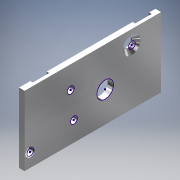
# Autodesk Inventor part: OslonaLewejPrzekladni
Saved by Autodesk Inventor 2019 (Build 230136000, 136)
## iProperties
Created: 2022-03-16
Part Number: OslonaLewejPrzekladni
Material: Aluminium 6061
Document SubType Name: Modeling
Designer: Michał
Density: 2.7 g/cm^3
Appearance: Aluminium — płaski
Mass: 6.40731 g
Surface Area: 27.93 cm^2
Volume: 2.37308 cm^3
Author: Michał
Autodesk Inventor part; units mm, degrees
ref_plane "YZ Plane" through (0, 0, 0) normal (1, 0, 0) x (0, 1, 0)
sketch "Szkic1" plane through (0, 0, 0) normal (1, 0, 0) x (0, 1, 0)
  line L0 (0, 0) -> (25, 0)
  line L1 (25, 0) -> (25, -49)
  line L2 (25, -49) -> (0, -49)
  line L3 (0, -49) -> (0, 0)
  dimension "d0" = 25
  dimension "d1" = 49
  constraints: 8 end point, 2 parallel, 1 horizontal, 1 perpendicular
  measures "d0" distance of L0.start L0.end
  measures "d1" distance of L0.end L1.end
extrude "Wyciągnięcie proste1" add sketch "Szkic1" along normal blind 2
sketch "Szkic2" plane through (2, 0, 0) normal (1, 0, 0) x (0, 0, -1)
  circle A0 centre (28.9, 11) radius 3
  circle A1 centre (17.6791, 7.0925) radius 1.25
  circle A2 centre (16.5416, 17.0276) radius 1.25
  circle A3 centre (2, 5) radius 1.2295
  circle A4 centre (38.5, 20) radius 1.2295
  constraints: 5 centre point, 10 other
hole "Otwór1" at (2, 5, -2) direction (-1, 0, 0) diameter 3.4 end through all clearance for "Śruba ze łbem stożkowym ISO 2009/7046" size "M3" standard "ISO"
hole "Otwór2" at (2, 20, -38.5) direction (-1, 0, 0) diameter 3.4 end through all countersink diameter 6.3 countersink angle 90 clearance for "Śruba ze łbem stożkowym ISO 2009/7046" size "M3" standard "ISO"
extrude "Wyciągnięcie proste2" cut sketch "Szkic2" against normal through all contours A0 | A1 | A2
sketch "Szkic3" plane through (0, 25, 0) normal (0, 1, 0) x (1, 0, 0)
  line L0 (0, 4.05) -> (-5, 4.05)
  line L1 (-5, 46.7) -> (0, 46.7)
  line L2 (0, 40.8) -> (-5, 40.8)
  line L3 (0, 4.05) -> (0.9, 4.05)
  line L4 (0.9, 4.05) -> (0.9, 9.95)
  line L5 (0.9, 9.95) -> (0, 9.95)
  line L6 (0, 9.95) -> (0, 4.05)
  line L7 (0, 40.8) -> (0.9, 40.8)
  line L8 (0.9, 40.8) -> (0.9, 46.7)
  line L9 (0.9, 46.7) -> (0, 46.7)
  line L10 (0, 46.7) -> (0, 40.8)
  dimension "d30" = 0.9
  constraints: 22 end point, 5 horizontal, 5 parallel, 2 equal length, 2 perpendicular, 1 collinear, 6 other
  measures "d30" distance of L0.start L3.end
ref_plane "Płaszczyzna konstrukcyjna1" through (-5, 2, -9.0505) normal (0, 1, 0) x (0, 0, 1)
ref_plane "Płaszczyzna konstrukcyjna2" through (-5, 2, -8.0505) normal (0, 1, 0) x (0, 0, 1)
extrude "Wyciągnięcie proste3" cut sketch "Szkic3" against normal up to surface (23 mm away)
fillet "Zaokrąglenie1" radius 1 4 edges at (0.45, 2, -40.8) (0.45, 2, -46.7) (0.45, 2, -9.95) (0.45, 2, -4.05)
